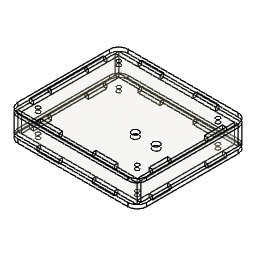
enclosure (Autodesk Fusion 360 design; units mm, degrees)
Autodesk Fusion 360 part; units mm, degrees
note: some values were not read from the file. Set by a fixed rule: which sketch regions a step uses.
sketch "Sketch1" plane through (0, 0, 0) normal (0, 0, 1) x (1, 0, 0) in component "Bottom"
  line L0 (5, 60) -> (65, 60)
  line L1 (70, 55) -> (70, 5)
  line L2 (65, 0) -> (5, 0)
  line L3 (0, 5) -> (0, 55)
  circle A0 centre (62, 52) radius 1.1
  line L4 (35, 60) -> (35, 0) construction
  line L5 (0, 30) -> (70, 30) construction
  circle A1 centre (8, 52) radius 1.1
  circle A2 centre (8, 8) radius 1.1
  circle A3 centre (62, 8) radius 1.1
  arc A4 (5, 60) -> (0, 55) centre (5, 55) ccw
  arc A5 (70, 55) -> (65, 60) centre (65, 55) ccw
  arc A6 (65, 0) -> (70, 5) centre (65, 5) ccw
  arc A7 (0, 5) -> (5, 0) centre (5, 5) ccw
  line L6 (5, 55) -> (65, 55) construction
  line L7 (5, 5) -> (5, 55) construction
  line L8 (65, 5) -> (5, 5) construction
  line L9 (65, 55) -> (65, 5) construction
  line L10 (66.5, 50) -> (68.5, 50)
  line L11 (68.5, 50) -> (68.5, 40)
  line L12 (68.5, 40) -> (66.5, 40)
  line L13 (66.5, 40) -> (66.5, 50)
  line L14 (70, 45) -> (0, 45) construction
  line L15 (70, 15) -> (0, 15) construction
  line L16 (3.5, 40) -> (3.5, 50)
  line L17 (3.5, 50) -> (1.5, 50)
  line L18 (1.5, 50) -> (1.5, 40)
  line L19 (1.5, 40) -> (3.5, 40)
  line L20 (1.5, 10) -> (1.5, 20)
  line L21 (3.5, 10) -> (1.5, 10)
  line L22 (3.5, 20) -> (3.5, 10)
  line L23 (1.5, 20) -> (3.5, 20)
  line L24 (66.5, 10) -> (68.5, 10)
  line L25 (66.5, 20) -> (66.5, 10)
  line L26 (68.5, 10) -> (68.5, 20)
  line L27 (68.5, 20) -> (66.5, 20)
  line L28 (20, 60) -> (20, 0) construction
  line L29 (14, 58.5) -> (26, 58.5)
  line L30 (26, 58.5) -> (26, 56.5)
  line L31 (26, 56.5) -> (14, 56.5)
  line L32 (14, 56.5) -> (14, 58.5)
  line L33 (50, 60) -> (50, 0) construction
  line L34 (56, 58.5) -> (44, 58.5)
  line L35 (56, 56.5) -> (56, 58.5)
  line L36 (44, 56.5) -> (56, 56.5)
  line L37 (44, 58.5) -> (44, 56.5)
  line L38 (14, 1.5) -> (26, 1.5)
  line L39 (14, 3.5) -> (14, 1.5)
  line L40 (26, 3.5) -> (14, 3.5)
  line L41 (26, 1.5) -> (26, 3.5)
  line L42 (56, 3.5) -> (56, 1.5)
  line L43 (56, 1.5) -> (44, 1.5)
  line L44 (44, 1.5) -> (44, 3.5)
  line L45 (44, 3.5) -> (56, 3.5)
  point P0 (0, 60)
  point P1 (70, 60)
  point P2 (70, 0)
  dimension "d4" = 70
  dimension "d5" = 60
  dimension "d6" = 2.2
  dimension "d7" = 8
  dimension "d8" = 8
  dimension "d9" = 5
  dimension "d10" = 5
  dimension "d16" = 2
  dimension "d17" = 10
  dimension "d19" = 1.5
  dimension "d20" = 15
  dimension "d22" = 5
  dimension "d23" = 15
  dimension "d24" = 12
  dimension "d25" = 2
  dimension "d26" = 1.5
  dimension "d27" = 6
  constraint horizontal L0
  constraint vertical L1
  constraint horizontal L2
  constraint vertical L3
  constraint symmetric A0 L4 A1
  constraint symmetric A0 L5 A3
  constraint symmetric L5 A1 A2
  constraint coincident L3 L5.start
  constraint coincident L0 L4.start
  constraint coincident P0 L3
  constraint coincident P0 L0
  constraint tangent L3 A4
  constraint tangent L0 A4
  constraint coincident L1 L5.end
  constraint coincident P1 L0
  constraint coincident P1 L1
  constraint tangent L0 A5
  constraint tangent L1 A5
  constraint equal A4 A5
  constraint coincident L2 L4.end
  constraint coincident P2 L1
  constraint coincident P2 L2
  constraint tangent L1 A6
  constraint tangent L2 A6
  constraint equal A4 A6
  constraint tangent L2 A7
  constraint tangent L3 A7
  constraint equal A4 A7
  constraint horizontal L10
  constraint vertical L11
  constraint horizontal L12
  constraint vertical L13
  constraint coincident L1 L14.start
  constraint coincident L3 L14.end
  constraint perpendicular L3 L14
  constraint symmetric L5 L14.start L15.start
  constraint symmetric L5 L14.end L15.end
  constraint symmetric L4 L10.start L16.end
  constraint symmetric L4 L10.end L17.end
  constraint symmetric L4 L11.end L18.end
  constraint symmetric L4 L12.end L16.start
  constraint symmetric L5 L10.start L24.start
  constraint symmetric L5 L10.end L24.end
  constraint symmetric L5 L11.end L26.end
  constraint symmetric L5 L12.end L25.start
  constraint symmetric L5 L16.start L22.start
  constraint symmetric L5 L16.end L21.start
  constraint symmetric L5 L17.end L20.start
  constraint symmetric L5 L18.end L20.end
  constraint coincident L0 L28.start
  constraint coincident L2 L28.end
  constraint perpendicular L2 L28
  constraint horizontal L29
  constraint vertical L30
  constraint horizontal L31
  constraint vertical L32
  constraint symmetric L4 L28.start L33.start
  constraint symmetric L4 L28.end L33.end
  constraint symmetric L4 L29.start L34.start
  constraint symmetric L4 L29.end L34.end
  constraint symmetric L4 L30.end L36.start
  constraint symmetric L4 L31.end L35.start
  constraint symmetric L5 L29.start L38.start
  constraint symmetric L5 L29.end L38.end
  constraint symmetric L5 L30.end L40.start
  constraint symmetric L5 L31.end L39.start
  constraint symmetric L5 L34.start L42.end
  constraint symmetric L5 L34.end L43.end
  constraint symmetric L5 L35.start L42.start
  constraint symmetric L5 L36.start L44.end
  measures "d4" distance of P0 P1
  measures "d5" distance of P1 P2
  measures "d6" diameter of A0
  measures "d7" distance of L0 A0.centre
  measures "d8" distance of L1 A0.centre
  measures "d9" radius of A4
  measures "d16" distance of L10.start L10.end
  measures "d17" distance of L10.end L11.end
  measures "d19" distance of L9 L13
  measures "d20" distance of L5 L14
  measures "d22" distance of L12 L14
  measures "d23" distance of L4 L28
  measures "d24" distance of L29.start L29.end
  measures "d25" distance of L29.start L31.end
  measures "d26" distance of L6 L31
  measures "d27" distance of L28 L32
extrude "Extrude2" add sketch "Sketch1" along normal blind 2 makes body 1 in component "Bottom"
sketch "Sketch1 (2)" plane through (1.5, 0, 0) normal (1, 0, 0) x (0, 1, 0) in component "Left"
  line L0 (10, 0) -> (20, 0)
  line L1 (20, 0) -> (20, 2)
  line L2 (10, 2) -> (10, 0)
  line L3 (10, 0) -> (10, 2)
  line L4 (40, 0) -> (40, 2)
  line L5 (20, 0) -> (20, 2)
  line L6 (50, 0) -> (50, 2)
  line L7 (3.5, 0) -> (3.5, 2) construction
  line L8 (56.5, 0) -> (56.5, 2) construction
  line L9 (20, 0) -> (10, 0)
  line L10 (40, 0) -> (50, 0)
  line L11 (40, 2) -> (20, 2)
  line L12 (50, 2) -> (56.5, 2)
  line L13 (3.5, 2) -> (10, 2)
  line L14 (56.5, 2) -> (56.5, 12.3)
  line L15 (3.5, 2) -> (3.5, 12.3)
  line L16 (56.5, 7.15) -> (3.5, 7.15) construction
  line L17 (3.5, 12.3) -> (10, 12.3)
  line L18 (10, 12.3) -> (10, 14.3)
  line L19 (20, 14.3) -> (10, 14.3)
  line L20 (20, 14.3) -> (20, 12.3)
  line L21 (40, 12.3) -> (20, 12.3)
  line L22 (40, 14.3) -> (40, 12.3)
  line L23 (40, 14.3) -> (50, 14.3)
  line L24 (50, 14.3) -> (50, 12.3)
  line L25 (50, 12.3) -> (56.5, 12.3)
  dimension "d30" = 10.3
  constraint coincident L0.end L1.start
  constraint coincident L0.start L2.end
  constraint coincident L4.start L10.start
  constraint coincident L6.start L10.end
  constraint coincident L4.end L11.start
  constraint coincident L1.end L5.end
  constraint coincident L6.end L12.start
  constraint coincident L8.end L12.end
  constraint coincident L7.end L13.start
  constraint coincident L2.start L3.end
  constraint perpendicular L12 L14
  constraint perpendicular L13 L15
  constraint midpoint L14 L16.start
  constraint midpoint L15 L16.end
  constraint symmetric L0.start L16 L18.end
  constraint symmetric L0.end L16 L19.start
  constraint symmetric L1.end L16 L20.end
  constraint symmetric L2.start L16 L17.end
  constraint symmetric L4.start L16 L22.start
  constraint symmetric L4.end L16 L21.start
  constraint symmetric L6.start L16 L23.end
  constraint symmetric L6.end L16 L24.end
  constraint symmetric L8.end L16 L14.end
  constraint symmetric L7.end L16 L15.end
  constraint coincident L15.end L17.start
  measures "d30" distance of L8.end L14.end
extrude "Extrude1" add sketch "Sketch1 (2)" along normal blind 2 separate body makes body 2 in component "Left"
sketch "Sketch1 (3)" plane through (66.5, 0, 0) normal (1, 0, 0) x (0, 1, 0) in component "Right"
  line L0 (10, 0) -> (20, 0)
  line L1 (20, 0) -> (20, 2)
  line L2 (10, 2) -> (10, 0)
  line L3 (40, 14.3) -> (50, 14.3)
  line L4 (50, 14.3) -> (50, 12.3)
  line L5 (50, 12.3) -> (56.5, 12.3)
  line L6 (56.5, 2) -> (56.5, 12.3)
  line L7 (50, 2) -> (56.5, 2)
  line L8 (50, 0) -> (50, 2)
  line L9 (40, 0) -> (50, 0)
  line L10 (40, 0) -> (40, 2)
  line L11 (40, 2) -> (20, 2)
  line L12 (20, 0) -> (20, 2)
  line L13 (20, 0) -> (10, 0)
  line L14 (10, 0) -> (10, 2)
  line L15 (3.5, 2) -> (10, 2)
  line L16 (3.5, 2) -> (3.5, 12.3)
  line L17 (3.5, 12.3) -> (10, 12.3)
  line L18 (10, 12.3) -> (10, 14.3)
  line L19 (20, 14.3) -> (10, 14.3)
  line L20 (20, 14.3) -> (20, 12.3)
  line L21 (40, 12.3) -> (20, 12.3)
  line L22 (40, 14.3) -> (40, 12.3)
extrude "Extrude1'" add sketch "Sketch1 (3)" along normal blind 2 separate body makes body 3 in component "Right"
sketch "Sketch1 (4)" plane through (0, 3.5, 0) normal (0, -1, 0) x (1, 0, 0) in component "Front"
  line L0 (14, 0) -> (26, 0)
  line L1 (26, 0) -> (26, 2)
  line L2 (14, 2) -> (14, 0)
  line L3 (1.5, 2) -> (1.5, 12.3)
  line L4 (68.5, 12.3) -> (68.5, 2)
  line L5 (26, 0) -> (26, 2)
  line L6 (56, 0) -> (56, 2)
  line L7 (14, 0) -> (14, 2)
  line L8 (44, 0) -> (44, 2)
  line L9 (1.5, 2) -> (14, 2)
  line L10 (14, 0) -> (26, 0)
  line L11 (26, 2) -> (44, 2)
  line L12 (44, 0) -> (56, 0)
  line L13 (56, 2) -> (68.5, 2)
  line L14 (68.5, 7.15) -> (1.5, 7.15) construction
  line L15 (1.5, 12.3) -> (14, 12.3)
  line L16 (14, 12.3) -> (14, 14.3)
  line L17 (14, 14.3) -> (26, 14.3)
  line L18 (26, 14.3) -> (26, 12.3)
  line L19 (26, 12.3) -> (44, 12.3)
  line L20 (44, 14.3) -> (44, 12.3)
  line L21 (44, 14.3) -> (56, 14.3)
  line L22 (56, 14.3) -> (56, 12.3)
  line L23 (56, 12.3) -> (68.5, 12.3)
  point P0 (44, 2)
  constraint coincident L3.start L9.start
  constraint coincident L2.start L7.end
  constraint coincident L0.start L2.end
  constraint coincident L0.end L1.start
  constraint coincident L1.end L5.end
  constraint coincident P0 L8.end
  constraint coincident L8.start L12.start
  constraint coincident L6.start L12.end
  constraint coincident L6.end L13.start
  constraint coincident L4.end L13.end
  constraint midpoint L4 L14.start
  constraint midpoint L3 L14.end
  constraint symmetric L0.start L14 L16.end
  constraint symmetric L0.end L14 L17.end
  constraint symmetric L1.end L14 L18.end
  constraint symmetric L2.start L14 L15.end
  constraint symmetric L6.start L14 L21.end
  constraint symmetric L6.end L14 L22.end
  constraint symmetric L8.start L14 L20.start
  constraint symmetric P0 L14 L19.end
  constraint symmetric L3.start L14 L3.end
  constraint symmetric L4.end L14 L4.start
extrude "Extrude1''" add sketch "Sketch1 (4)" along normal blind 2 separate body makes body 4 in component "Front"
sketch "Sketch2" plane through (0, 56.5, 0) normal (0, 1, 0) x (-1, 0, 0) in component "Back"
  line L0 (-56, 0) -> (-44, 0)
  line L1 (-44, 0) -> (-44, 2)
  line L2 (-56, 2) -> (-56, 0)
  line L3 (-56, 14.3) -> (-44, 14.3)
  line L4 (-56, 12.3) -> (-56, 14.3)
  line L5 (-68.5, 12.3) -> (-56, 12.3)
  line L6 (-68.5, 2) -> (-68.5, 12.3)
  line L7 (-56, 2) -> (-68.5, 2)
  line L8 (-56, 0) -> (-56, 2)
  line L9 (-44, 0) -> (-56, 0)
  line L10 (-44, 2) -> (-44, 0)
  line L11 (-26, 2) -> (-44, 2)
  line L12 (-26, 0) -> (-26, 2)
  line L13 (-14, 0) -> (-26, 0)
  line L14 (-14, 2) -> (-14, 0)
  line L15 (-1.5, 2) -> (-14, 2)
  line L16 (-1.5, 12.3) -> (-1.5, 2)
  line L17 (-14, 12.3) -> (-1.5, 12.3)
  line L18 (-14, 14.3) -> (-14, 12.3)
  line L19 (-26, 14.3) -> (-14, 14.3)
  line L20 (-26, 12.3) -> (-26, 14.3)
  line L21 (-44, 12.3) -> (-26, 12.3)
  line L22 (-44, 14.3) -> (-44, 12.3)
extrude "Extrude2'" add sketch "Sketch2" along normal blind 2 separate body makes body 5 in component "Back"
sketch "Sketch1 (5)" plane through (0, 0, 12.3) normal (0, 0, 1) x (-1, 0, 0) in component "Top"
  line L0 (-1.5, -40) -> (-1.5, -20)
  line L1 (-1.5, -20) -> (-3.5, -20)
  line L2 (-3.5, -20) -> (-3.5, -40)
  line L3 (-3.5, -40) -> (-1.5, -40)
  circle A0 centre (-8, -52) radius 1.1
  circle A1 centre (-62, -52) radius 1.1
  line L4 (-56, -1.5) -> (-44, -1.5)
  line L5 (-56, -3.5) -> (-56, -1.5)
  line L6 (-44, -3.5) -> (-56, -3.5)
  line L7 (-44, -1.5) -> (-44, -3.5)
  line L8 (-14, -3.5) -> (-26, -3.5)
  line L9 (-14, -1.5) -> (-14, -3.5)
  line L10 (-26, -1.5) -> (-14, -1.5)
  line L11 (-26, -3.5) -> (-26, -1.5)
  line L12 (-56, -56.5) -> (-44, -56.5)
  line L13 (-56, -58.5) -> (-56, -56.5)
  line L14 (-44, -58.5) -> (-56, -58.5)
  line L15 (-44, -56.5) -> (-44, -58.5)
  line L16 (-26, -58.5) -> (-26, -56.5)
  line L17 (-14, -58.5) -> (-26, -58.5)
  line L18 (-14, -56.5) -> (-14, -58.5)
  line L19 (-26, -56.5) -> (-14, -56.5)
  line L20 (-66.5, -10) -> (-66.5, -20)
  line L21 (-68.5, -10) -> (-66.5, -10)
  line L22 (-68.5, -20) -> (-68.5, -10)
  line L23 (-66.5, -20) -> (-68.5, -20)
  line L24 (-3.5, -10) -> (-1.5, -10)
  line L25 (-3.5, -20) -> (-3.5, -10)
  line L26 (-1.5, -20) -> (-3.5, -20)
  line L27 (-1.5, -10) -> (-1.5, -20)
  line L28 (-3.5, -50) -> (-3.5, -40)
  line L29 (-1.5, -50) -> (-3.5, -50)
  line L30 (-1.5, -40) -> (-1.5, -50)
  line L31 (-3.5, -40) -> (-1.5, -40)
  line L32 (-68.5, -50) -> (-68.5, -40)
  line L33 (-66.5, -50) -> (-68.5, -50)
  line L34 (-66.5, -40) -> (-66.5, -50)
  line L35 (-68.5, -40) -> (-66.5, -40)
  circle A2 centre (-62, -8) radius 1.1
  circle A3 centre (-8, -8) radius 1.1
  line L36 (-5, -60) -> (-65, -60)
  arc A4 (-70, -55) -> (-65, -60) centre (-65, -55) ccw
  line L37 (-70, -55) -> (-70, -5)
  arc A5 (-65, 0) -> (-70, -5) centre (-65, -5) ccw
  line L38 (-65, 0) -> (-5, 0)
  arc A6 (0, -5) -> (-5, 0) centre (-5, -5) ccw
  line L39 (0, -5) -> (0, -55)
  arc A7 (-5, -60) -> (0, -55) centre (-5, -55) ccw
extrude "Extrude1'''" add sketch "Sketch1 (5)" along normal blind 2 separate body makes body 6 in component "Top"
sketch "Sketch2 (2)" plane through (0, 0, 14.3) normal (0, 0, 1) x (-1, 0, 0) in component "Top"
  circle A0 centre (-8, -8) radius 1.1
  line L0 (-68.5, -50) -> (-68.5, -40)
  line L1 (-68.5, -40) -> (-66.5, -40)
  line L2 (-66.5, -40) -> (-66.5, -50)
  line L3 (-66.5, -50) -> (-68.5, -50)
  circle A1 centre (-8, -52) radius 1.1
  line L4 (-3.5, -50) -> (-3.5, -10)
  line L5 (-3.5, -10) -> (-1.5, -10)
  line L6 (-1.5, -10) -> (-1.5, -50)
  line L7 (-1.5, -50) -> (-3.5, -50)
  line L8 (-66.5, -10) -> (-66.5, -20)
  line L9 (-66.5, -20) -> (-68.5, -20)
  line L10 (-68.5, -20) -> (-68.5, -10)
  line L11 (-68.5, -10) -> (-66.5, -10)
  circle A2 centre (-62, -8) radius 1.1
  line L12 (-26, -58.5) -> (-26, -56.5)
  line L13 (-26, -56.5) -> (-14, -56.5)
  line L14 (-14, -56.5) -> (-14, -58.5)
  line L15 (-14, -58.5) -> (-26, -58.5)
  line L16 (-56, -56.5) -> (-44, -56.5)
  line L17 (-44, -56.5) -> (-44, -58.5)
  line L18 (-44, -58.5) -> (-56, -58.5)
  line L19 (-56, -58.5) -> (-56, -56.5)
  line L20 (-14, -3.5) -> (-26, -3.5)
  line L21 (-26, -3.5) -> (-26, -1.5)
  line L22 (-26, -1.5) -> (-14, -1.5)
  line L23 (-14, -1.5) -> (-14, -3.5)
  circle A3 centre (-62, -52) radius 1.1
  line L24 (-56, -1.5) -> (-44, -1.5)
  line L25 (-44, -1.5) -> (-44, -3.5)
  line L26 (-44, -3.5) -> (-56, -3.5)
  line L27 (-56, -3.5) -> (-56, -1.5)
  arc A4 (-70, -55) -> (-65, -60) centre (-65, -55) ccw
  line L28 (-65, -60) -> (-5, -60)
  arc A5 (-5, -60) -> (0, -55) centre (-5, -55) ccw
  line L29 (0, -55) -> (0, -5)
  arc A6 (0, -5) -> (-5, 0) centre (-5, -5) ccw
  line L30 (-5, 0) -> (-65, 0)
  arc A7 (-65, 0) -> (-70, -5) centre (-65, -5) ccw
  line L31 (-70, -5) -> (-70, -55)
  circle A8 centre (-46.2, -22.8) radius 1.9
  circle A9 centre (-57.4, -22.9) radius 1.9
  dimension "d50" = 3.8
  dimension "d51" = 3.8
  measures "d50" diameter of A8
  measures "d51" diameter of A9
extrude "Extrude2''" cut sketch "Sketch2 (2)" against normal up to surface (2 mm away) contours A8 | A9 bodies 6 in component "Top"
component "Bottom" placed x (1, 0, 0) y (0, 1, 0) z (0, 0, 1) at (0, 0, 0)
component "Left" placed x (1, 0, 0) y (0, 1, 0) z (0, 0, 1) at (0, 0, 0)
component "Right" placed x (1, 0, 0) y (0, 1, 0) z (0, 0, 1) at (0, 0, 0)
component "Front" placed x (1, 0, 0) y (0, 1, 0) z (0, 0, 1) at (0, 0, 0)
component "Back" placed x (1, 0, 0) y (0, 1, 0) z (0, 0, 1) at (0, 0, 0)
component "Top" placed x (1, 0, 0) y (0, 1, 0) z (0, 0, 1) at (0, 0, 0)
equation "paddingLength = 5 mm"
equation "filletRadius = 5 mm"
equation "mountingHoleDiameter = 3.2 mm"
equation "d4 = 60 mm + 2 * paddingLength"
equation "d5 = 50 mm + 2 * paddingLength"
equation "d7 = 3 mm + paddingLength"
equation "d8 = 3 mm + paddingLength"
equation "d9 = filletRadius"
equation "d10 = paddingLength"
equation "thickness = 2 mm"
equation "tabLength = 10 mm"
equation "tabWidth = 2 mm"
equation "d16 = tabWidth"
equation "d17 = tabLength"
equation "d22 = tabLength / 2"
equation "d24 = tabLength * 1.2"
equation "d25 = tabWidth"
equation "d27 = ( tabLength * 1.2 ) / 2"
equation "d28 = thickness"
equation "d30 = 3.7 mm + 1.6 mm + 3.8 mm + 1.2 mm"
equation "d31 = tabWidth"
equation "d33 = tabWidth"
equation "d35 = tabWidth"
equation "d39 = tabWidth"
equation "d48 = thickness"
